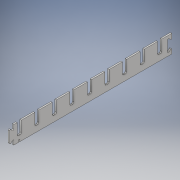
# Autodesk Inventor part: PLASMA TEMPLATE CUTTING
Saved by Autodesk Inventor 2019 (Build 230136000, 136)
## iProperties
Created: 2019-03-12
Part Number: PLASMA TEMPLATE CUTTING
Material: Generic
Document SubType Name: Modeling
Designer: torba
Density: 1 g/cm^3
Appearance: Default
Author: torba
Autodesk Inventor part; units mm, degrees
ref_plane "YZ Plane" through (0, 0, 0) normal (1, 0, 0) x (0, 1, 0)
ref_plane "XZ Plane" through (0, 0, 0) normal (0, 1, 0) x (-1, 0, 0)
ref_plane "XY Plane" through (0, 0, 0) normal (0, 0, 1) x (1, 0, 0)
sketch "Sketch1" plane through (0, 0, 0) normal (1, 0, 0) x (0, 1, 0)
  line L0 (0, 0) -> (25.4, 0)
  line L1 (76.2, 675.9763) -> (0, 675.9763)
  line L2 (0, 675.9763) -> (0, 0)
  line L3 (76.2, 655.1416) -> (31.75, 655.1416) construction
  line L4 (31.75, 655.1416) -> (31.75, 650.3791) construction
  line L5 (31.75, 650.3791) -> (76.2, 650.3791) construction
  line L6 (76.2, 650.3791) -> (76.2, 655.1416) construction
  line L7 (76.2, 661.6026) -> (30.75, 661.6026)
  line L8 (25.289, 656.1416) -> (25.289, 649.3791)
  line L9 (30.75, 643.9181) -> (76.2, 643.9181)
  line L10 (76.2, 643.9181) -> (76.2, 661.6026)
  arc A0 (30.75, 661.6026) -> (25.289, 656.1416) centre (30.75, 656.1416) ccw
  arc A1 (25.289, 649.3791) -> (30.75, 643.9181) centre (30.75, 649.3791) ccw
  line L11 (76.2, 0) -> (50.8, 0)
  line L12 (0, 0) -> (25.4, 0)
  line L13 (25.4, 0) -> (7.4395, 17.9605)
  line L14 (50.8, 0) -> (68.7605, 17.9605)
  line L15 (68.7605, 17.9605) -> (7.4395, 17.9605)
  line L16 (76.2, 675.9763) -> (58.4651, 675.9763)
  line L17 (0, 675.9763) -> (25.4, 675.9763)
  line L18 (76.2, 675.9763) -> (50.8, 675.9763)
  line L19 (50.8, 675.9763) -> (68.7605, 693.9368)
  line L20 (0, 675.9763) -> (25.4, 675.9763)
  line L21 (25.4, 675.9763) -> (7.4395, 693.9368)
  line L22 (68.7605, 693.9368) -> (7.4395, 693.9368)
  line L23 (76.2, 675.9763) -> (76.2, 0)
  line L24 (50.8, 675.9763) -> (25.4, 675.9763)
  line L25 (50.8, 675.9763) -> (25.4, 675.9763)
  line L26 (76.2, 568.8103) -> (76.2, 586.4948)
  line L27 (30.75, 568.8103) -> (76.2, 568.8103)
  line L28 (76.2, 586.4948) -> (30.75, 586.4948)
  arc A2 (30.75, 586.4948) -> (25.289, 581.0338) centre (30.75, 581.0338) ccw
  arc A3 (25.289, 574.2713) -> (30.75, 568.8103) centre (30.75, 574.2713) ccw
  line L29 (25.289, 581.0338) -> (25.289, 574.2713)
  line L30 (76.2, 493.7025) -> (76.2, 511.387)
  line L31 (30.75, 493.7025) -> (76.2, 493.7025)
  line L32 (76.2, 511.387) -> (30.75, 511.387)
  arc A4 (30.75, 511.387) -> (25.289, 505.926) centre (30.75, 505.926) ccw
  arc A5 (25.289, 499.1635) -> (30.75, 493.7025) centre (30.75, 499.1635) ccw
  line L33 (25.289, 505.926) -> (25.289, 499.1635)
  line L34 (76.2, 418.5947) -> (76.2, 436.2792)
  line L35 (30.75, 418.5947) -> (76.2, 418.5947)
  line L36 (76.2, 436.2792) -> (30.75, 436.2792)
  arc A6 (30.75, 436.2792) -> (25.289, 430.8182) centre (30.75, 430.8182) ccw
  arc A7 (25.289, 424.0557) -> (30.75, 418.5947) centre (30.75, 424.0557) ccw
  line L37 (25.289, 430.8182) -> (25.289, 424.0557)
  line L38 (76.2, 343.4869) -> (76.2, 361.1714)
  line L39 (30.75, 343.4869) -> (76.2, 343.4869)
  line L40 (76.2, 361.1714) -> (30.75, 361.1714)
  arc A8 (30.75, 361.1714) -> (25.289, 355.7104) centre (30.75, 355.7104) ccw
  arc A9 (25.289, 348.9479) -> (30.75, 343.4869) centre (30.75, 348.9479) ccw
  line L41 (25.289, 355.7104) -> (25.289, 348.9479)
  line L42 (76.2, 268.3791) -> (76.2, 286.0636)
  line L43 (30.75, 268.3791) -> (76.2, 268.3791)
  line L44 (76.2, 286.0636) -> (30.75, 286.0636)
  arc A10 (30.75, 286.0636) -> (25.289, 280.6026) centre (30.75, 280.6026) ccw
  arc A11 (25.289, 273.8401) -> (30.75, 268.3791) centre (30.75, 273.8401) ccw
  line L45 (25.289, 280.6026) -> (25.289, 273.8401)
  line L46 (76.2, 193.2713) -> (76.2, 210.9558)
  line L47 (30.75, 193.2713) -> (76.2, 193.2713)
  line L48 (76.2, 210.9558) -> (30.75, 210.9558)
  arc A12 (30.75, 210.9558) -> (25.289, 205.4948) centre (30.75, 205.4948) ccw
  arc A13 (25.289, 198.7323) -> (30.75, 193.2713) centre (30.75, 198.7323) ccw
  line L49 (25.289, 205.4948) -> (25.289, 198.7323)
  line L50 (76.2, 118.1635) -> (76.2, 135.848)
  line L51 (30.75, 118.1635) -> (76.2, 118.1635)
  line L52 (76.2, 135.848) -> (30.75, 135.848)
  arc A14 (30.75, 135.848) -> (25.289, 130.387) centre (30.75, 130.387) ccw
  arc A15 (25.289, 123.6245) -> (30.75, 118.1635) centre (30.75, 123.6245) ccw
  line L53 (25.289, 130.387) -> (25.289, 123.6245)
  line L54 (76.2, 43.0557) -> (76.2, 60.7402)
  line L55 (30.75, 43.0557) -> (76.2, 43.0557)
  line L56 (76.2, 60.7402) -> (30.75, 60.7402)
  arc A16 (30.75, 60.7402) -> (25.289, 55.2792) centre (30.75, 55.2792) ccw
  arc A17 (25.289, 48.5167) -> (30.75, 43.0557) centre (30.75, 48.5167) ccw
  line L57 (25.289, 55.2792) -> (25.289, 48.5167)
  line L58 (31.75, 655.1416) -> (0, 655.1416)
  line L59 (0, 655.1416) -> (0, 650.3664)
  line L60 (0, 650.3664) -> (31.75, 650.3664)
  line L61 (31.75, 650.3664) -> (31.75, 655.1416)
  line L62 (0, 655.1416) -> (9.525, 655.1416)
  line L63 (9.525, 655.1416) -> (9.525, 650.3664)
  line L64 (9.525, 650.3664) -> (0, 650.3664)
  line L65 (0, 650.3664) -> (0, 655.1416)
  point P0 (50.8, 0)
  point P1 (7.4395, 17.9605)
  point P2 (68.7605, 17.9605)
  point P3 (25.4, 0)
  point P4 (50.8, 0)
  dimension "d21" = 0
  dimension "d0" = 76.2
  dimension "d3" = 4.7625
  dimension "d5" = 6.461
  dimension "d6" = 6.461
  dimension "d7" = 6.461
  dimension "d8" = 5.461
  dimension "d16" = 25.4
  dimension "d17" = 25.4
  dimension "d18" = 25.4
  dimension "d19" = 45
  dimension "d20" = 25.4
  dimension "d28" = 25.4
  dimension "d29" = 25.4
  dimension "d30" = 45
  dimension "d31" = 25.4
  dimension "d32" = 25.4
  dimension "d33" = 45
  dimension "d34" = 32.3342
  dimension "d36" = 0
  dimension "d37" = 44.45
  dimension "d38" = 76.2
  dimension "d40" = 17.7349
  dimension "d47" = 75.1078
  dimension "d52" = 25.0952
  dimension "d55" = 9.525
  dimension "d59" = 4.7752
  constraints: 132 end point, 36 point on circle, 18 centre point, 13 point on line, 12 parallel, 11 horizontal, 5 perpendicular, 4 tangent, 2 collinear, 1 equal radius, 1 vertical, 132 other
  measures "d0" distance of L1.end L1.start
  measures "d3" distance of L4.end L3.end
  measures "d5" distance between parallel lines of L4 L8
  measures "d6" distance between parallel lines of L7 L3
  measures "d7" distance between parallel lines of L9 L5
  measures "d8" radius of A0
  measures "d16" distance of L11.start point (50.8, 0)
  measures "d17" distance of L0.start L12.end
  measures "d18" distance of L12.end point (7.439, 17.961)
  measures "d19" angle of L13 L12
  measures "d20" distance of point (50.8, 0) point (68.761, 17.961)
  measures "d28" distance of L16.start L18.end
  measures "d29" distance of L18.end L19.end
  measures "d30" angle of L18 L19
  measures "d31" distance of L17.start L17.end
  measures "d32" distance of L17.end L21.end
  measures "d33" angle of L21 L20
  measures "d34" distance between parallel lines of L7 L22
  measures "d36" distance between parallel lines of L6 L23
  measures "d37" distance between parallel lines of L6 L4
  measures "d38" distance between parallel lines of L6 L2
  measures "d40" distance from line of L16.end L6
  measures "d47" distance of L9.end L26.start
  measures "d52" distance between parallel lines of L55 L15
  measures "d55" distance of L63.end L64.end
  measures "d59" distance between parallel lines of L60 L58
extrude "Extrusion3" add sketch "Sketch1" along normal blind 6.35 contours L2 L60 L8 A1 L9 L23 L28 A2 L29 A3 L27 L32 A4 L33 A5 L31 L36 A6 L37 A7 L35 L40 A8 L41 A9 L39 L44 A10 L45 A11 L43 L48 A12 L49 A13 L47 L52 A14 L53 A15 L51 L56 A16 L57 A17 L55 L11 L14 L15 L13 L0 | L2 L58 L63 L60 | L2 L1 L23 L7 A0 L8 L58 | L63 L58 L8 L60 | L21 L22 L19 L1
extrude "Extrusion4" cut sketch "Sketch1" along normal blind 6.35 contours L2 L58 L63 L60
fillet "Fillet1" radius 3.175 8 edges at (3.175, 7.4395, 693.9368) (3.175, 25.4, 675.9763) (3.175, 50.8, 675.9763) (3.175, 68.7605, 693.9368) (3.175, 68.7605, 17.9605) (3.175, 7.4395, 17.9605) (3.175, 50.8, 0) (3.175, 25.4, 0)
equation "\"d6\" = d5"
equation "\"d7\" = d6"
body "Solid2"
